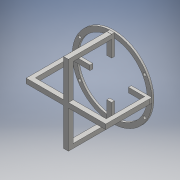
# Autodesk Inventor part: Bottom- Control Surfaces
Saved by Autodesk Inventor 2016 (Build 200138000, 138)
## iProperties
Created: 2016-03-15
Part Number: Bottom- Control Surfaces
Material: Generic
Document SubType Name: Modeling
Designer: s_sud
Density: 1 g/cm^3
Appearance: Default
Author: s_sud
Autodesk Inventor part; units mm, degrees
ref_plane "YZ Plane" through (0, 0, 0) normal (1, 0, 0) x (0, 1, 0)
ref_plane "XZ Plane" through (0, 0, 0) normal (0, 1, 0) x (-1, 0, 0)
ref_plane "XY Plane" through (0, 0, 0) normal (0, 0, 1) x (1, 0, 0)
sketch "Sketch1" plane through (0, 0, 0) normal (0, 1, 0) x (-1, 0, 0)
  circle A0 centre (0, 0) radius 41.5
  circle A1 centre (0, 0) radius 36.5
  dimension "d0" = 83
  dimension "d1" = 73
  constraints: 2 centre point, 2 coincident
  measures "d0" diameter of A0
  measures "d1" diameter of A1
extrude "Extrusion1" add sketch "Sketch1" along normal blind 2
sketch "Sketch4" plane through (0, 0, 0) normal (0, -1, 0) x (1, 0, 0)
  line L0 (-2.5, -20) -> (-2.5, -41.5)
  line L1 (-2.5, -41.5) -> (2.5, -41.5)
  line L2 (2.5, -41.5) -> (2.5, -20)
  line L3 (3.2204, 53.4593) -> (-2.5, -41.5) construction
  line L4 (-3.2204, 53.4593) -> (2.5, -41.5) construction
  line L5 (2.5, -20) -> (-2.5, -20)
  line L6 (41.5, 2.5) -> (20, 2.5)
  line L7 (20, -2.5) -> (41.5, -2.5)
  line L8 (20, 2.5) -> (20, -2.5)
  line L9 (41.5, -2.5) -> (41.5, 2.5)
  line L10 (-2.5, 41.5) -> (-2.5, 20)
  line L11 (2.5, 20) -> (2.5, 41.5)
  line L12 (-2.5, 20) -> (2.5, 20)
  line L13 (2.5, 41.5) -> (-2.5, 41.5)
  line L14 (-41.5, -2.5) -> (-20, -2.5)
  line L15 (-20, 2.5) -> (-41.5, 2.5)
  line L16 (-20, -2.5) -> (-20, 2.5)
  line L17 (-41.5, 2.5) -> (-41.5, -2.5)
  point P0 (0, 0)
  dimension "d21" = 5
  dimension "d26" = 360
  dimension "d51" = 20
  dimension "d52" = 41.5
  constraints: 36 end point, 2 point on line, 1 parallel, 1 perpendicular, 33 other
  measures "d21" distance of L0.end L1.end
  measures "d51" distance from line of L5 point (0, 0)
  measures "d52" distance from line of point (0, 0) L1
extrude "Extrusion3" add sketch "Sketch4" along normal blind 3
sketch "Sketch5" plane through (0, -3, 0) normal (0, -1, 0) x (1, 0, 0)
  arc A0 (-41.4246, 2.5) -> (2.5, -41.4246) centre (0, 0) ccw projected
  line L0 (2.5, -41.4246) -> (-2.5, -41.4246)
  line L1 (-2.5, -41.4246) -> (-2.5, -36.9246)
  line L2 (-2.5, -36.9246) -> (2.5, -36.9246)
  line L3 (2.5, -36.9246) -> (2.5, -41.4246)
  line L4 (41.4246, 2.5) -> (41.4246, -2.5)
  line L5 (41.4246, -2.5) -> (36.9246, -2.5)
  line L6 (36.9246, -2.5) -> (36.9246, 2.5)
  line L7 (36.9246, 2.5) -> (41.4246, 2.5)
  line L8 (-2.5, 41.4246) -> (2.5, 41.4246)
  line L9 (2.5, 41.4246) -> (2.5, 36.9246)
  line L10 (2.5, 36.9246) -> (-2.5, 36.9246)
  line L11 (-2.5, 36.9246) -> (-2.5, 41.4246)
  line L12 (-41.4246, -2.5) -> (-41.4246, 2.5)
  line L13 (-41.4246, 2.5) -> (-36.9246, 2.5)
  line L14 (-36.9246, 2.5) -> (-36.9246, -2.5)
  line L15 (-36.9246, -2.5) -> (-41.4246, -2.5)
  point P0 (0, -41.5)
  dimension "d30" = 5
  dimension "d31" = 4.5
  dimension "d34" = 360
  constraints: 32 end point, 2 parallel, 1 horizontal, 1 perpendicular, 33 other
  measures "d30" distance of L1.end L2.end
  measures "d31" distance of L0.end L1.end
extrude "Extrusion4" add sketch "Sketch5" along normal blind 40 contours L13 L14 L15 L12 | L1 L2 L3 L0 | L4 L5 L6 L7 | L8 L9 L10 L11
sketch "Sketch7" plane through (0, 2, 0) normal (0, 1, 0) x (1, 0, 0)
  circle A0 centre (0, -39) radius 1.5
  circle A1 centre (0, -44.5) radius 1.5
  circle A2 centre (38.5381, -22.25) radius 1.5
  circle A3 centre (33.775, -19.5) radius 1.5
  circle A4 centre (38.5381, 22.25) radius 1.5
  circle A5 centre (33.775, 19.5) radius 1.5
  circle A6 centre (0, 44.5) radius 1.5
  circle A7 centre (0, 39) radius 1.5
  circle A8 centre (-38.5381, 22.25) radius 1.5
  circle A9 centre (-33.775, 19.5) radius 1.5
  circle A10 centre (-38.5381, -22.25) radius 1.5
  circle A11 centre (-33.775, -19.5) radius 1.5
  point P0 (0, 0)
  dimension "d41" = 3
  dimension "d42" = 39
  dimension "d43" = 3
  dimension "d44" = 44.5
  dimension "d47" = 360
  constraints: 12 centre point, 25 other
  measures "d41" diameter of A0
  measures "d42" distance of point (0, 0) A0.centre
  measures "d43" diameter of A1
  measures "d44" distance of point (0, 0) A1.centre
extrude "Extrusion6" cut sketch "Sketch7" against normal blind 10 contours A2 | A3 | A4 | A5 | A8 | A9 | A10 | A11
sketch "Sketch8" plane through (0, -43, 0) normal (0, -1, 0) x (1, 0, 0)
  line L0 (-2.5, 36.4143) -> (-2.5, 41.4246) projected
  arc A0 (0, -41.5) -> (2.5, -41.4246) centre (0, 0) ccw projected
  line L1 (-2.5, 41.4246) -> (2.5, 41.4246)
  line L2 (2.5, 41.4246) -> (2.5, -41.4246)
  line L3 (2.5, -41.4246) -> (-2.5, -41.4246)
  line L4 (-2.5, -41.4246) -> (-2.5, 41.4246)
  line L5 (-36.4143, -2.5) -> (-41.4246, -2.5) projected
  line L6 (36.4143, 2.5) -> (41.4246, 2.5) projected
  line L7 (-41.4246, -2.5) -> (41.4246, -2.5)
  line L8 (41.4246, -2.5) -> (41.4246, 2.5)
  line L9 (41.4246, 2.5) -> (-41.4246, 2.5)
  line L10 (-41.4246, 2.5) -> (-41.4246, -2.5)
  constraints: 16 end point, 4 parallel, 2 horizontal, 2 perpendicular
extrude "Extrusion7" add sketch "Sketch8" along normal blind 5
body "Solid1"
